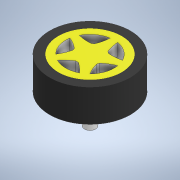
# Autodesk Inventor part: mock_wheel
Saved by Autodesk Inventor 2020.3 (Build 243373000, 373)
## iProperties
Created: 2020-07-03
Part Number: mock_wheel
Material: Generic
Document SubType Name: Modeling
Designer: Devin
Density: 1 g/cm^3
Appearance: Default
Author: Devin
Autodesk Inventor part; units mm, degrees
ref_plane "YZ Plane" through (0, 0, 0) normal (1, 0, 0) x (0, 1, 0)
ref_plane "XZ Plane" through (0, 0, 0) normal (0, 1, 0) x (-1, 0, 0)
ref_plane "XY Plane" through (0, 0, 0) normal (0, 0, 1) x (1, 0, 0)
sketch "Sketch1" plane through (0, 0, 0) normal (0, 1, 0) x (-1, 0, 0)
  circle A0 centre (0, 0) radius 32.5
  circle A1 centre (0, 0) radius 25.5
  dimension "d0" = 65
  dimension "d1" = 51
  constraints: 2 centre point, 2 coincident
  measures "d0" diameter of A0
  measures "d1" diameter of A1
extrude "Extrusion1" add sketch "Sketch1" along normal blind 26
sketch "Sketch2" plane through (0, 26, 0) normal (0, 1, 0) x (1, 0, 0)
  circle A0 centre (0, 0) radius 9
  arc A1 (-5.4083, 9) -> (-3.0109, 19.2661) centre (-32.5925, 20.7613) ccw
  arc A2 (3.0109, 19.2661) -> (5.4083, 9) centre (32.5925, 20.7613) ccw
  arc A3 (-10.2308, -2.3625) -> (-19.2536, 3.09) centre (-29.8168, -24.5817) ccw
  arc A4 (-17.3928, 8.8171) -> (-6.8882, 7.9248) centre (-9.6735, 37.4129) ccw
  arc A5 (-0.9146, -10.4601) -> (-8.8885, -17.3564) centre (14.1647, -35.9536) ccw
  arc A6 (-13.7602, -13.8169) -> (-9.6655, -4.1022) centre (-38.5711, 2.3612) ccw
  arc A7 (9.6655, -4.1022) -> (13.7602, -13.8169) centre (38.5711, 2.3612) ccw
  arc A8 (8.8885, -17.3564) -> (0.9146, -10.4601) centre (-14.1647, -35.9536) ccw
  arc A9 (6.8882, 7.9248) -> (17.3928, 8.8171) centre (9.6735, 37.4129) ccw
  arc A10 (19.2536, 3.09) -> (10.2308, -2.3625) centre (29.8168, -24.5817) ccw
  arc A11 (-3.0109, 19.2661) -> (-17.3928, 8.8171) centre (0, 0) ccw
  arc A12 (-19.2536, 3.09) -> (-13.7602, -13.8169) centre (0, 0) ccw
  arc A13 (-8.8885, -17.3564) -> (8.8885, -17.3564) centre (0, 0) ccw
  arc A14 (13.7602, -13.8169) -> (19.2536, 3.09) centre (0, 0) ccw
  arc A15 (17.3928, 8.8171) -> (3.0109, 19.2661) centre (0, 0) ccw
  arc A16 (-5.4083, 9) -> (-6.8882, 7.9248) centre (0, 0) ccw
  arc A17 (-10.2308, -2.3625) -> (-9.6655, -4.1022) centre (0, 0) ccw
  arc A18 (-0.9146, -10.4601) -> (0.9146, -10.4601) centre (0, 0) ccw
  arc A19 (9.6655, -4.1022) -> (10.2308, -2.3625) centre (0, 0) ccw
  arc A20 (6.8882, 7.9248) -> (5.4083, 9) centre (0, 0) ccw
  circle A21 centre (0, 0) radius 25.45
  circle A22 centre (0, 0) radius 19.5
  point P0 (-17.3928, 8.8171)
  point P1 (-19.2536, 3.09)
  point P2 (-8.8885, -17.3564)
  point P3 (8.8885, -17.3564)
  point P4 (13.7602, -13.8169)
  point P5 (19.2536, 3.09)
  point P6 (17.3928, 8.8171)
  point P7 (-3.0109, 19.2661)
  dimension "d6" = 18
  dimension "d11" = 360
  dimension "d15" = 50.9
  constraints: 40 point on circle, 23 centre point, 5 coincident, 41 other
  measures "d6" diameter of A0
  measures "d15" diameter of A21
extrude "Extrusion3" add sketch "Sketch2" against normal blind 10 contours A1 A22 A2 A20 A9 A10 A19 A7 A8 A18 A5 A6 A17 A3 A4 A16
sketch "Sketch3" plane through (0, 26, 0) normal (0, 1, 0) x (1, 0, 0)
  arc A0 (-17.3928, 8.8171) -> (-19.2536, 3.09) centre (0, 0) ccw projected
  circle A1 centre (0, 0) radius 19.5
  circle A2 centre (0, 0) radius 25.495
  point P0 (-17.3928, 8.8171)
  dimension "d18" = 50.99
  constraints: 2 coincident, 1 centre point, 3 other
  measures "d18" diameter of A2
extrude "Extrusion4" add sketch "Sketch3" against normal up to surface (26 mm away)
sketch "Sketch4" plane through (0, 26, 0) normal (0, 1, 0) x (1, 0, 0)
  circle A0 centre (0, 0) radius 9
  constraints: 1 centre point, 1 coincident
extrude "Extrusion5" add sketch "Sketch4" against normal blind 15
sketch "Sketch5" plane through (0, 11, 0) normal (0, -1, 0) x (1, 0, 0)
  circle A0 centre (0, 0) radius 2
  circle A1 centre (0, 0) radius 4.5
  dimension "d23" = 4
  dimension "d24" = 9
  constraints: 2 centre point, 2 coincident
  measures "d23" diameter of A0
  measures "d24" diameter of A1
extrude "Extrusion6" add sketch "Sketch5" along normal blind 35
body "Solid1"
